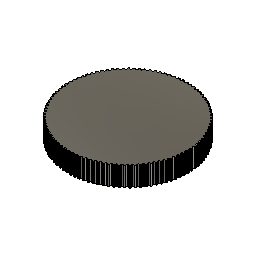
gear_97z (Autodesk Fusion 360 design; units mm, degrees)
Autodesk Fusion 360 part; units mm, degrees
sketch "Sketch1" plane through (0, 0, 0) normal (0, 0, 1) x (1, 0, 0) in component "gt2 pulley"
  circle A0 centre (0, 0) radius 30.8761 construction
  circle A1 centre (0, 0) radius 29.8721 construction
  line L0 (0, 0) -> (0, 30.8761) construction
  line L1 (0, 0) -> (0.9998, 30.8599) construction
  line L2 (0, 0) -> (1.4041, 30.8441) construction
  circle A2 centre (0, 0) radius 30.6221 construction
  arc A3 (0.398, 30.4866) -> (0.4773, 30.1875) centre (1.3926, 30.5904) ccw
  circle A4 centre (0, 0) radius 30.4721 construction
  arc A5 (0.2499, 30.621) -> (0, 30.6221) centre (0, 0) ccw
  arc A6 (0.398, 30.4866) -> (0.2499, 30.621) centre (0.2488, 30.471) ccw
  arc A7 (0.4773, 30.1875) -> (0.9673, 29.8564) centre (0.9853, 30.4111) ccw
  arc A8 (0, 30.6221) -> (-0.2499, 30.621) centre (0, 0) ccw
  arc A9 (-0.2499, 30.621) -> (-0.398, 30.4866) centre (-0.2488, 30.471) ccw
  arc A10 (-0.4773, 30.1875) -> (-0.398, 30.4866) centre (-1.3926, 30.5904) ccw
  arc A11 (-0.9676, 29.8564) -> (-0.4773, 30.1875) centre (-0.9853, 30.4111) ccw
  arc A12 (0.9673, 29.8564) -> (-0.9673, 29.8564) centre (0, 0) ccw
  point P0 (1.3926, 30.5904)
  point P1 (0, 30.6221)
  dimension "d18" = 61.7521
  dimension "d19" = 1.856
  dimension "d22" = 1.004
  dimension "d24" = 0.75
  dimension "d26" = 1
  dimension "d27" = 0.15
  dimension "d28" = 0.15
  dimension "d47" = 0.555
  dimension "d52" = 3.812
  constraint coincident A0.centre A1.centre
  constraint coincident A0 L0.end
  constraint vertical L0
  constraint coincident A0 L1.end
  constraint coincident A0 L2.end
  constraint concentric A1 A2
  constraint coincident A1 A7.end
  constraint coincident L1 A7.end
  constraint coincident A2 P0
  constraint coincident L2 P0
  constraint coincident P0 A3.centre
  constraint coincident A2 P1
  constraint coincident L0 P1
  constraint concentric A2 A4
  constraint coincident P1 A5.end
  constraint coincident A4 A6.centre
  constraint coincident A3.start A6.start
  constraint tangent A3 A6
  constraint tangent A3 A7
  constraint symmetric L0 A7.end A12.end
  constraint symmetric L0 A3.start A9.end
  constraint symmetric L0 A3.end A10.start
  constraint symmetric L0 A3 A10
  constraint symmetric L0 A5.start A8.end
  constraint symmetric L0 P1 A5.end
  constraint symmetric L0 A5 A8
  constraint symmetric L0 A6 A9
  constraint symmetric L0 A7 A11
  constraint coincident A1 A11.start
  constraint tangent A1 A7
  constraint coincident L1 A7.centre
  measures "d18" diameter of A0
  measures "d19" angle of L0 L1
  measures "d22" distance of A0 A1
  measures "d24" distance of A1 A2
  measures "d26" radius of A3
  measures "d27" distance of A2 A4
  measures "d28" radius of A6
  measures "d47" radius of A7
extrude "Extrude1" add sketch "Sketch1" along normal blind 10 makes body 1
pattern_circular "C-Pattern1" count 97 over 360 about axis through (0, 0, 1.75) along (0, 0, 1) of bodies 1 makes body 2 at (-1.8264, 29.8162, 6.6667) makes body 3 at (-3.9658, 29.6076, 6.6667) makes body 4 at (-5.874, 29.2888, 6.6667) makes body 5 at (-6.9239, 29.0586, 3.3333) makes body 6 at (-8.7903, 28.5494, 3.3333) makes body 7 at (-11.4193, 27.6033, 6.6667) makes body 8 at (-13.7578, 26.5153, 6.6667) makes body 9 at (-14.8896, 25.8967, 6.6667) makes body 10 at (-16.5346, 24.8786, 6.6667) makes body 11 at (-17.4189, 24.2677, 6.6667) makes body 12 at (-18.9533, 23.0893, 6.6667) makes body 13 at (-20.4081, 21.814, 6.6667) makes body 14 at (-21.7773, 20.4472, 3.3333) makes body 15 at (-23.5924, 18.3231, 6.6667) makes body 16 at (-24.2363, 17.4625, 6.6667) makes body 17 at (-25.7619, 15.1217, 6.6667) makes body 18 at (-26.9703, 12.8431, 6.6667) makes body 19 at (-27.1523, 12.4537, 6.6667) makes body 20 at (-28.3361, 9.4554, 6.6667) makes body 21 at (-28.7763, 8.0165, 6.6667) makes body 22 at (-29.0461, 6.9761, 3.3333) makes body 23 at (-29.4367, 5.0813, 3.3333) makes body 24 at (-29.7039, 3.1652, 3.3333) makes body 25 at (-29.8697, 0.3761, 6.6667) makes body 26 at (-29.8418, -1.3434, 6.6667) makes body 27 at (-29.756, -2.6303, 3.3333) makes body 28 at (-29.2993, -5.8213, 6.6667) makes body 29 at (-28.969, -7.2894, 6.6667) makes body 30 at (-28.688, -8.3268, 3.3333) makes body 31 at (-27.5412, -11.5682, 6.6667) makes body 32 at (-27.3719, -11.9632, 3.3333) makes body 33 at (-25.8159, -15.0292, 6.6667) makes body 34 at (-24.789, -16.6688, 6.6667) makes body 35 at (-24.5466, -17.0237, 3.3333) makes body 36 at (-23.3931, -18.5769, 3.3333) makes body 37 at (-22.1416, -20.0522, 6.6667) makes body 38 at (-20.3293, -21.8874, 6.6667) makes body 39 at (-19.3656, -22.7446, 3.3333) makes body 40 at (-17.8527, -23.9504, 3.3333) makes body 41 at (-14.9824, -25.8432, 6.6667) makes body 42 at (-13.2781, -26.7588, 6.6667) makes body 43 at (-12.8918, -26.947, 3.3333) makes body 44 at (-10.3177, -28.0337, 6.6667) makes body 45 at (-9.3025, -28.3867, 3.3333) makes body 46 at (-7.4455, -28.9293, 3.3333) makes body 47 at (-5.5573, -29.3506, 3.3333) makes body 48 at (-3.6458, -29.6487, 3.3333) makes body 49 at (-1.719, -29.8226, 3.3333) makes body 50 at (1.0749, -29.8527, 6.6667) makes body 51 at (3.005, -29.7205, 6.6667) makes body 52 at (4.9225, -29.4637, 6.6667) makes body 53 at (5.9793, -29.2675, 3.3333) makes body 54 at (7.8612, -28.8191, 3.3333) makes body 55 at (11.1207, -27.7249, 6.6667) makes body 56 at (12.892, -26.9469, 6.6667) makes body 57 at (14.6092, -26.0559, 6.6667) makes body 58 at (14.9826, -25.843, 3.3333) makes body 59 at (17.8529, -23.9502, 6.6667) makes body 60 at (18.1956, -23.6909, 3.3333) makes body 61 at (20.7974, -21.4432, 6.6667) makes body 62 at (21.9969, -20.2108, 6.6667) makes body 63 at (23.3933, -18.5767, 6.6667) makes body 64 at (24.1734, -17.5495, 6.6667) makes body 65 at (25.5972, -15.3989, 6.6667) makes body 66 at (26.5402, -13.7097, 6.6667) makes body 67 at (26.7347, -13.3264, 3.3333) makes body 68 at (27.5413, -11.5679, 3.3333) makes body 69 at (28.6881, -8.3266, 6.6667) makes body 70 at (29.0208, -7.0805, 6.6667) makes body 71 at (29.2567, -6.0319, 3.3333) makes body 72 at (29.7561, -2.6301, 6.6667) makes body 73 at (29.8418, -1.3431, 6.6667) makes body 74 at (29.8709, -0.2687, 3.3333) makes body 75 at (29.8256, 1.6654, 3.3333) makes body 76 at (29.5395, 4.4447, 6.6667) makes body 77 at (29.2348, 6.1372, 6.6667) makes body 78 at (28.7178, 8.2237, 6.6667) makes body 79 at (28.4034, 9.2514, 3.3333) makes body 80 at (27.7449, 11.0706, 6.6667) makes body 81 at (26.2891, 14.1854, 6.6667) makes body 82 at (25.3157, 15.8573, 6.6667) makes body 83 at (24.3613, 17.2878, 6.6667) makes body 84 at (23.4598, 18.4927, 6.6667) makes body 85 at (22.2136, 19.9724, 6.6667) makes body 86 at (20.4079, 21.8142, 6.6667) makes body 87 at (20.0919, 22.1055, 6.6667) makes body 88 at (18.1102, 23.7563, 6.6667) makes body 89 at (15.8114, 25.3444, 6.6667) makes body 90 at (14.1377, 26.3148, 6.6667) makes body 91 at (12.9885, 26.9005, 6.6667) makes body 92 at (10.6196, 27.9207, 6.6667) makes body 93 at (10.2168, 28.0706, 3.3333) makes body 94 at (7.5495, 28.9023, 6.6667) makes body 95 at (5.8738, 29.2889, 6.6667) makes body 96 at (3.9656, 29.6077, 6.6667) makes body 97 at (1.8262, 29.8162, 6.6667)
sketch "Sketch2" plane through (0, 0, 10) normal (0, 0, 1) x (-1, 0, 0)
  arc A0 (-8.1957, -29.367) -> (-8.0871, -29.5349) centre (-8.0475, -29.3902) ccw
  arc A1 (-8.0871, -29.5349) -> (-7.6038, -29.663) centre (0, 0) ccw
  arc A2 (-7.6038, -29.663) -> (-7.4263, -29.571) centre (-7.5665, -29.5177) ccw
  arc A3 (-7.273, -29.3022) -> (-7.4263, -29.571) centre (-6.4915, -29.9261) ccw
  arc A4 (-6.7145, -29.1076) -> (-7.273, -29.3022) centre (-6.8393, -29.6484) ccw
  arc A5 (-8.5846, -28.612) -> (-6.7145, -29.1076) centre (0, 0) ccw
  arc A6 (-8.1958, -29.0576) -> (-8.5846, -28.612) centre (-8.7441, -29.1436) ccw
  arc A7 (-8.1957, -29.367) -> (-8.1958, -29.0576) centre (-9.1837, -29.2125) ccw
  circle A8 centre (0, 0) radius 29.8721
  constraint coincident A1.centre A5.centre
extrude "Extrude2" add sketch "Sketch2" against normal blind 10 contours A5 A8 bodies 1 2 3 4 5 6 7 8 9 10 11 12 13 14 15 16 17 18 19 20 21 22 23 24 25 26 27 28 29 30 31 32 33 34 35 36 37 38 39 40 41 42 43 44 45 46 47 48 49 50 51 52 53 54 55 56 57 58 59 60 61 62 63 64 65 66 67 68 69 70 71 72 73 74 75 76 77 78 79 80 81 82 83 84 85 86 87 88 89 90 91 92 93 94 95 96 97
extrude "Extrude4" [suppressed] in component "gt2 pulley"
pattern_circular "C-Pattern7" [suppressed] in component "gt2 pulley"
extrude "Extrude3" [suppressed] in component "gt2 pulley"
pattern_circular "C-Pattern6" [suppressed] in component "gt2 pulley"
extrude "Extrude2'" [suppressed] in component "gt2 pulley"
pattern_circular "C-Pattern5" [suppressed] in component "gt2 pulley"
extrude "Extrude1'" [suppressed] in component "gt2 pulley"
pattern_circular "C-Pattern4" [suppressed] in component "gt2 pulley"
pattern_circular "C-Pattern3" [suppressed] in component "gt2 pulley"
pattern_circular "C-Pattern2" [suppressed] in component "gt2 pulley"
pattern_circular "C-Pattern1'" [suppressed] in component "gt2 pulley"
copy_body "Body->Comp1" [suppressed] in component "Component"
copy_body "Body->Comp2" [suppressed] in component "Component'"
copy_body "Body->Comp3" [suppressed] in component "Component''"
copy_body "Body->Comp4" [suppressed] in component "Component'''"
copy_body "Body->Comp5" [suppressed] in component "Component''''"
copy_body "Body->Comp6" [suppressed] in component "Component'''''"
copy_body "Body->Comp7" [suppressed] in component "Component''''''"
copy_body "Body->Comp8" [suppressed] in component "Component'''''''"
copy_body "Body->Comp9" [suppressed] in component "Component''''''''"
copy_body "Body->Comp10" [suppressed] in component "Component'''''''''"
copy_body "Body->Comp11" [suppressed] in component "Component''''''''''"
copy_body "Body->Comp12" [suppressed] in component "Component'''''''''''"
copy_body "Body->Comp13" [suppressed] in component "Component''''''''''''"
copy_body "Body->Comp14" [suppressed] in component "Component'''''''''''''"
copy_body "Body->Comp15" [suppressed] in component "Component''''''''''''''"
copy_body "Body->Comp16" [suppressed] in component "Component'''''''''''''''"
copy_body "Body->Comp17" [suppressed] in component "Component''''''''''''''''"
copy_body "Body->Comp18" [suppressed] in component "Component'''''''''''''''''"
copy_body "Body->Comp19" [suppressed] in component "Component''''''''''''''''''"
copy_body "Body->Comp20" [suppressed] in component "Component'''''''''''''''''''"
component "gt2 pulley" placed x (1, 0, 0) y (0, 1, 0) z (0, 0, 1) at (0, 0, 0)
equation "NumTeeth = 97" comment "min 20"
equation "ToothPitch = 2 mm"
equation "PullyDia = NumTeeth * ToothPitch / PI"
equation "ToothAng = ( ( 360 / NumTeeth ) * 1 deg )"
equation "TransOffsetAngle = ToothAng * 0.2"
equation "Sholulder_Radius = 0.15 mm"
equation "Root_Radius = 0.555 mm"
equation "TransRadius = 1 mm"
equation "ToolHeight = 0.75 mm"
equation "PLD = 0.254 mm"
equation "d18 = PullyDia"
equation "d19 = ToothAng / 2"
equation "d22 = PLD + ToolHeight"
equation "d24 = ToolHeight"
equation "d26 = TransRadius"
equation "d27 = Sholulder_Radius"
equation "d31 = NumTeeth"
equation "d33 = NumTeeth"
equation "d35 = NumTeeth"
equation "d37 = NumTeeth"
equation "d41 = NumTeeth"
equation "d45 = NumTeeth"
equation "d47 = Root_Radius"
equation "d50 = NumTeeth"
